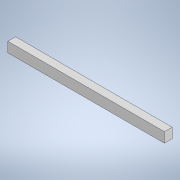
# Autodesk Inventor part: slider
Saved by Autodesk Inventor 2022 (Build 260153000, 153)
## iProperties
Created: 2022-05-17
Part Number: slider
Material: Generic
Document SubType Name: Sheet Metal
Designer: joshn
Density: 1 g/cm^3
Sheet Metal Rule: Default
Appearance: Default
Author: joshn
Autodesk Inventor part; units mm, degrees
ref_plane "YZ Plane" through (0, 0, 0) normal (1, 0, 0) x (0, 1, 0)
ref_plane "XZ Plane" through (0, 0, 0) normal (0, 1, 0) x (-1, 0, 0)
ref_plane "XY Plane" through (0, 0, 0) normal (0, 0, 1) x (1, 0, 0)
sketch "Sketch3" plane through (0, 0, 0) normal (0, 0, 1) x (1, 0, 0)
  line L0 (-39.7021, -77.224) -> (-9.3521, -77.224)
  line L1 (-9.3521, -77.224) -> (-9.3521, -75.274)
  line L2 (-9.3521, -75.274) -> (-39.7021, -75.274)
  line L3 (-39.7021, -75.274) -> (-39.7021, -77.224)
  point P0 (0, 0)
  dimension "d3" = 30.35
  dimension "d4" = 1.95
  measures "d3" distance of L2.end L1.end
  measures "d4" distance of L1.end L0.end
extrude "Plate1" add sketch "Sketch3" along normal blind 1.5
equation "\"d5\" = Thickness"
equation "\"BendRadius\" = Thickness"
equation "\"BendReliefWidth\" = Thickness"
equation "\"BendReliefDepth\" = 0.5 * Thickness"
equation "\"CornerReliefSize\" = 4 * Thickness"
equation "\"MinimumRemnant\" = 2 * Thickness"
equation "\"TransitionRadius\" = BendRadius"
equation "\"JacobiRadiusSize\" = BendRadius"
equation "\"GapSize\" = Thickness"
equation "\"Thickness\" = 1.5"
body "Solid1"
